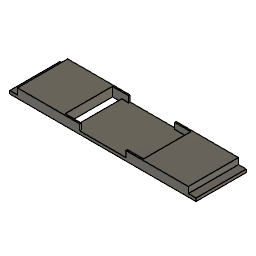
Canal - middle plate v4 (Autodesk Fusion 360 design; units mm, degrees)
Autodesk Fusion 360 part; units mm, degrees
sketch "Esquisse1" plane through (0, 0, 0) normal (0, 0, 1) x (1, 0, 0)
  line L0 (9.4, 40) -> (70, 40)
  line L1 (70, 40) -> (70, 23.65)
  line L2 (70, 23.65) -> (9.4, 23.65)
  line L3 (9.4, 23.65) -> (9.4, 40)
  dimension "d1" = 60.6
  dimension "d2" = 16.35
  constraint horizontal L0
  constraint vertical L1
  constraint horizontal L2
  constraint vertical L3
  measures "d1" distance of L1 L3
  measures "d2" distance of L0 L2
extrude "Extrusion1" add sketch "Esquisse1" along normal blind 3
sketch "Esquisse2" plane through (0, 0, 0) normal (0, 0, -1) x (1, 0, 0)
  line L0 (70, -23.65) -> (9.4, -23.65)
  line L1 (9.4, -23.65) -> (9.4, -40)
  line L2 (9.4, -40) -> (70, -40)
  line L3 (70, -40) -> (70, -23.65)
  line L4 (17.1, -25.55) -> (22.3, -25.55)
  line L5 (22.3, -25.55) -> (22.3, -27.75)
  line L6 (22.3, -27.75) -> (17.1, -27.75)
  line L7 (17.1, -27.75) -> (17.1, -25.55)
  line L8 (19.7, -25.55) -> (19.7, -27.75) construction
  line L9 (39.7, -23.65) -> (39.7, -40) construction
  line L10 (57.1, -25.55) -> (57.1, -27.75)
  line L11 (62.3, -25.55) -> (57.1, -25.55)
  line L12 (62.3, -27.75) -> (62.3, -25.55)
  line L13 (57.1, -27.75) -> (62.3, -27.75)
  line L14 (9.4, -31.825) -> (70, -31.825) construction
  line L15 (17.1, -38.1) -> (22.3, -38.1)
  line L16 (22.3, -38.1) -> (22.3, -35.9)
  line L17 (22.3, -35.9) -> (17.1, -35.9)
  line L18 (17.1, -35.9) -> (17.1, -38.1)
  line L19 (62.3, -38.1) -> (57.1, -38.1)
  line L20 (62.3, -35.9) -> (62.3, -38.1)
  line L21 (57.1, -35.9) -> (62.3, -35.9)
  line L22 (57.1, -38.1) -> (57.1, -35.9)
  dimension "d5" = 20
  dimension "d12" = 5.2
  dimension "d13" = 2.2
  dimension "d14" = 1.9
  constraint horizontal L4
  constraint vertical L5
  constraint horizontal L6
  constraint vertical L7
  constraint midpoint L4 L8.start
  constraint midpoint L6 L8.end
  constraint midpoint L0 L9.start
  constraint midpoint L2 L9.end
  constraint symmetric L4.start L9 L11.start
  constraint symmetric L4.end L9 L10.start
  constraint symmetric L5.end L9 L10.end
  constraint symmetric L6.end L9 L12.start
  constraint midpoint L1 L14.start
  constraint midpoint L3 L14.end
  constraint symmetric L4.start L14 L15.start
  constraint symmetric L4.end L14 L15.end
  constraint symmetric L5.end L14 L16.end
  constraint symmetric L6.end L14 L17.end
  constraint symmetric L10.start L14 L19.end
  constraint symmetric L10.end L14 L21.start
  constraint symmetric L11.start L14 L19.start
  constraint symmetric L12.start L14 L20.start
  measures "d5" distance of L8 L9
  measures "d12" distance of L5 L7
  measures "d13" distance of L4 L6
  measures "d14" distance of L0 L4
extrude "Extrusion2" cut sketch "Esquisse2" against normal blind 2 contours L4 L5 L6 L7 | L10 L11 L12 L13 | L15 L16 L17 L18 | L19 L20 L21 L22
sketch "Esquisse3" plane through (0, 0, 3) normal (0, 0, 1) x (-1, 0, 0)
  line L0 (-9.4, -23.65) -> (-70, -23.65)
  line L1 (-70, -23.65) -> (-70, -40)
  line L2 (-70, -40) -> (-9.4, -40)
  line L3 (-9.4, -40) -> (-9.4, -23.65)
  line L4 (-26.95, -39.525) -> (-52.45, -39.525)
  line L5 (-52.45, -39.525) -> (-52.45, -24.125)
  line L6 (-52.45, -24.125) -> (-26.95, -24.125)
  line L7 (-26.95, -24.125) -> (-26.95, -39.525)
  line L8 (-9.4, -31.825) -> (-70, -31.825) construction
  line L9 (-39.7, -40) -> (-39.7, -23.65) construction
  dimension "d8" = 25.5
  dimension "d9" = 15.4
  constraint horizontal L4
  constraint vertical L5
  constraint horizontal L6
  constraint vertical L7
  constraint midpoint L3 L8.start
  constraint midpoint L1 L8.end
  constraint midpoint L2 L9.start
  constraint midpoint L0 L9.end
  constraint symmetric L5 L7 L9
  constraint symmetric L0 L2 L8
  constraint symmetric L4 L6 L8
  measures "d8" distance of L5 L7
  measures "d9" distance of L4 L6
extrude "Extrusion3" cut sketch "Esquisse3" against normal blind 2 contours L4 L5 L6 L7
sketch "Esquisse4" plane through (0, 0, 1) normal (0, 0, 1) x (-1, 0, 0)
  line L0 (-26.95, -24.125) -> (-52.45, -24.125)
  line L1 (-52.45, -24.125) -> (-52.45, -39.525)
  line L2 (-52.45, -39.525) -> (-26.95, -39.525)
  line L3 (-26.95, -39.525) -> (-26.95, -24.125)
  line L4 (-26.95, -24.125) -> (-29.95, -24.125)
  line L5 (-29.95, -24.125) -> (-29.95, -39.525)
  line L6 (-29.95, -39.525) -> (-26.95, -39.525)
  line L7 (-26.95, -39.525) -> (-26.95, -24.125)
  dimension "d15" = 3
  constraint horizontal L4
  constraint vertical L5
  constraint horizontal L6
  constraint vertical L7
  constraint coincident L2 L5.end
  constraint coincident L0.start L3.end
  measures "d15" distance of L5 L7
extrude "Extrusion4" cut sketch "Esquisse4" against normal blind 3 contours L0 L2 L3 L4 L5 L6 L7
sketch "Esquisse5" plane through (0, 40, 0) normal (0, 1, 0) x (-1, 0, 0)
  line L0 (-70, 0) -> (-9.4, 0)
  line L1 (-9.4, 0) -> (-9.4, 3)
  line L2 (-9.4, 3) -> (-70, 3)
  line L3 (-70, 3) -> (-70, 0)
  line L4 (-39.7, 3) -> (-39.7, 0) construction
  line L5 (-47.2, 3) -> (-32.2, 3)
  line L6 (-32.2, 3) -> (-32.2, 1)
  line L7 (-32.2, 1) -> (-47.2, 1)
  line L8 (-47.2, 1) -> (-47.2, 3)
  dimension "d18" = 15
  dimension "d19" = 2
  constraint midpoint L2 L4.start
  constraint midpoint L0 L4.end
  constraint horizontal L5
  constraint vertical L6
  constraint horizontal L7
  constraint vertical L8
  constraint coincident L2 L5.start
  constraint symmetric L4 L6 L8
  measures "d18" distance of L6 L8
  measures "d19" distance of L5 L7
extrude "Extrusion5" cut sketch "Esquisse5" against normal blind 21 contours L2 L5 L6 L7 L8
sketch "Esquisse6" plane through (0, 0, 3) normal (0, 0, 1) x (-1, 0, 0)
  line L0 (-47.2, -24.125) -> (-47.2, -23.65)
  line L1 (-47.2, -23.65) -> (-70, -23.65)
  line L2 (-70, -23.65) -> (-70, -40)
  line L3 (-70, -40) -> (-47.2, -40)
  line L4 (-47.2, -40) -> (-47.2, -39.525)
  line L5 (-47.2, -39.525) -> (-52.45, -39.525)
  line L6 (-52.45, -39.525) -> (-52.45, -24.125)
  line L7 (-52.45, -24.125) -> (-47.2, -24.125)
  line L8 (-70, -40) -> (-67.5, -40)
  line L9 (-67.5, -40) -> (-67.5, -23.65)
  line L10 (-67.5, -23.65) -> (-70, -23.65)
  line L11 (-70, -23.65) -> (-70, -40)
  line L12 (-39.7, -39) -> (-39.7, -18) construction
  line L13 (-9.4, -23.65) -> (-9.4, -40)
  line L14 (-11.9, -23.65) -> (-9.4, -23.65)
  line L15 (-11.9, -40) -> (-11.9, -23.65)
  line L16 (-9.4, -40) -> (-11.9, -40)
  dimension "d22" = 2.5
  dimension "d23" = 30.3
  constraint horizontal L8
  constraint vertical L9
  constraint horizontal L10
  constraint vertical L11
  constraint coincident L1 L9.end
  constraint coincident L2.end L3.start
  constraint parallel L6 L12
  constraint symmetric L2.end L12 L13.end
  constraint symmetric L8.end L12 L15.start
  constraint symmetric L9.end L12 L14.start
  constraint symmetric L1.end L12 L13.start
  measures "d22" distance of L9 L11
  measures "d23" distance of L11 L12
extrude "Extrusion6" cut sketch "Esquisse6" against normal blind 2 contours L1 L2 L3 L8 L9 L10 L11 | L13 L14 L15 L16
